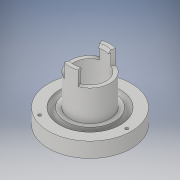
# Autodesk Inventor part: Blower Attachement
Saved by Autodesk Inventor 2019 (Build 230136000, 136)
## iProperties
Created: 2019-07-31
Part Number: Blower Attachement
Material: Generic
Document SubType Name: Modeling
Designer: Kepler
Density: 1 g/cm^3
Appearance: Default
Author: Kepler
Autodesk Inventor part; units mm, degrees
ref_plane "YZ Plane" through (0, 0, 0) normal (1, 0, 0) x (0, 1, 0)
ref_plane "XZ Plane" through (0, 0, 0) normal (0, 1, 0) x (-1, 0, 0)
ref_plane "XY Plane" through (0, 0, 0) normal (0, 0, 1) x (1, 0, 0)
sketch "Sketch1" plane through (0, 0, 0) normal (0, 1, 0) x (-1, 0, 0)
  circle A0 centre (0, 0) radius 21.5
  circle A1 centre (0, 0) radius 55
  dimension "d0" = 43
  dimension "d1" = 110
  constraints: 2 centre point, 2 coincident
  measures "d0" diameter of A0
  measures "d1" diameter of A1
extrude "Extrusion1" add sketch "Sketch1" along normal blind 20
sketch "Sketch2" plane through (0, 0, 0) normal (0, 0, 1) x (1, 0, 0)
  line L0 (0, 0) -> (0, 20)
  line L1 (55, 20) -> (-55, 20) projected
  circle A0 centre (-36.5, 17) radius 5
  line L2 (-21.5, 0) -> (-21.5, 20) construction
  line L3 (-21.5, 20) -> (-21.5, 0) construction
  dimension "d4" = 10
  dimension "d5" = 15
  constraints: 4 end point, 3 point on line, 1 centre point, 1 midpoint
  measures "d4" diameter of A0
  measures "d5" distance from line of A0.centre L2
revolve "Revolution1" cut sketch "Sketch2" angle 360 about axis through (0, 0, 0) along (0, 1, 0)
sketch "Sketch3" plane through (0, 20, 0) normal (0, 1, 0) x (1, 0, 0)
  circle A0 centre (0, 0) radius 21.5
  circle A1 centre (0, 0) radius 26.5
  circle A2 centre (0, 0) radius 21.5 projected
  dimension "d18" = 43
  dimension "d19" = 43
  dimension "d20" = 53
  constraints: 2 centre point, 2 coincident
  measures "d18" diameter of A2
  measures "d19" diameter of A0
  measures "d20" diameter of A1
extrude "Extrusion2" add sketch "Sketch3" along normal blind 60
sketch "Sketch4" plane through (0, 0, 0) normal (1, 0, 0) x (0, 1, 0)
  line L0 (80, 21.5) -> (80, -21.5) projected
  line L1 (80, -21.5) -> (76, -19)
  line L2 (76, -19) -> (76, -21.5)
  line L3 (0, -21.5) -> (80, -21.5) projected
  line L4 (80, -21.5) -> (76, -21.5)
  line L5 (80, 0) -> (74, 0)
  point P0 (0, 0)
  dimension "d9" = 2.5
  constraints: 8 end point, 1 midpoint, 1 perpendicular, 1 point on line, 1 vertical
  measures "d9" distance of L1.end L2.end
revolve "Revolution2" add sketch "Sketch4" angle 360 about axis through (0, 80, 0) along (0, -1, 0)
sketch "Sketch5" plane through (0, 80, 0) normal (0, 1, 0) x (1, 0, 0)
  line L0 (0, 4) -> (0, -4)
  line L1 (0, 0) -> (6.4984, 17.8542) construction
  line L2 (0, 0) -> (-6.4984, 17.8542) construction
  line L3 (0, 0) -> (9.0635, 24.9019) construction
  line L4 (0, 0) -> (0, 0) construction
  circle A0 centre (0, 0) radius 26.5 projected
  arc A1 (-9.0635, 24.9019) -> (-9.0635, -24.9019) centre (0, 0) ccw
  line L5 (0, 0) -> (-9.0635, -24.9019) construction
  line L6 (0, 0) -> (-9.0635, 24.9019) construction
  arc A2 (9.0635, -24.9019) -> (9.0635, 24.9019) centre (0, 0) ccw
  line L7 (0, 0) -> (9.0635, -24.9019) construction
  line L8 (0, 0) -> (9.0635, 24.9019) construction
  circle A3 centre (0, 0) radius 19 projected
  arc A4 (-6.4984, 17.8542) -> (-6.4984, -17.8542) centre (0, 0) ccw
  arc A5 (6.4984, -17.8542) -> (6.4984, 17.8542) centre (0, 0) ccw
  line L9 (-9.0635, -24.9019) -> (-6.4984, -17.8542)
  line L10 (6.4984, -17.8542) -> (9.0635, -24.9019)
  line L11 (6.4984, 17.8542) -> (9.0635, 24.9019)
  line L12 (-6.4984, 17.8542) -> (-9.0635, 24.9019)
  dimension "d22" = 40
  dimension "d23" = 40
  dimension "d24" = 20
  dimension "d25" = 20
  dimension "d26" = 140
  dimension "d27" = 140
  constraints: 26 end point, 10 point on circle, 6 coincident, 4 centre point, 4 collinear, 3 point on line, 1 vertical, 2 other
  measures "d22" angle of L1 L2
  measures "d23" angle of L3 L4
  measures "d26" angle of L6 L5
  measures "d27" angle of L7 L8
extrude "Extrusion3" cut sketch "Sketch5" against normal blind 19 contours A0 L10 A3 L11 | L12 A3 L9 A0
sketch "Sketch6" plane through (0, 0, 0) normal (0, -1, 0) x (1, 0, 0)
  circle A0 centre (49, 0) radius 2
  circle A1 centre (-24.5, 42.4352) radius 2
  circle A2 centre (-24.5, -42.4352) radius 2
  point P0 (0, 0)
  dimension "d32" = 360
  constraints: 3 centre point, 7 other
extrude "Extrusion4" cut sketch "Sketch6" against normal up to surface (20 mm away)
equation "\"d19\" = d18"
body "Solid1"
